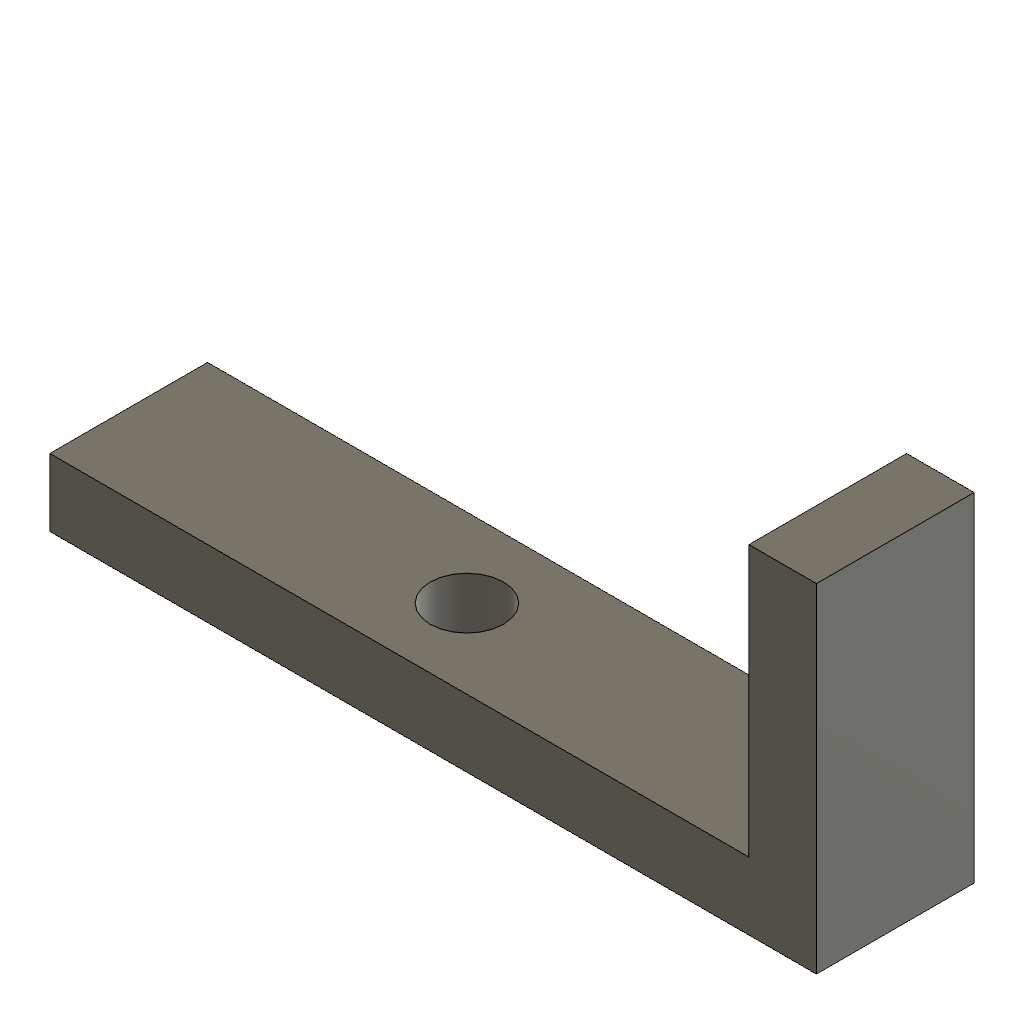
TankBot Ultrasonic Mount 2of2 (Autodesk Fusion 360 design; units mm, degrees)
Autodesk Fusion 360 part; units mm, degrees
box "BoxPrimitive1" add length 7 width 30 height 3 placed x (0, 0, 1) y (1, 0, 0) z (0, 1, 0) at (0, 0, 0)
hole "Hole1" at (15, 3, 3.5) direction (0, -1, 0) diameter 3.25 depth 3 tip angle 180
extrude "Extrude1" add 1 faces at (30, 1, 4.6667) along direction (1, 0, 0) blind 4
box "BoxPrimitive2" add length 7 width 3 height 12 placed x (0, 0, -1) y (-1, 0, 0) z (0, 1, 0) at (34, 3, 7)
